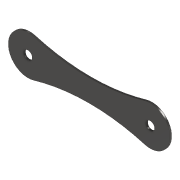
# Autodesk Inventor part: stelscharnier bovenkant
Saved by Autodesk Inventor 2020.3 (Build 243373000, 373)
## iProperties
Created: 2020-09-15
Part Number: stelscharnier bovenkant
Material: Stainless Steel
Document SubType Name: Modeling
Designer: Svend
Density: 8 g/cm^3
Appearance: Semi-Polished
Author: Svend
Autodesk Inventor part; units mm, degrees
ref_plane "YZ Plane" through (0, 0, 0) normal (1, 0, 0) x (0, 1, 0)
ref_plane "XZ Plane" through (0, 0, 0) normal (0, 1, 0) x (-1, 0, 0)
ref_plane "XY Plane" through (0, 0, 0) normal (0, 0, 1) x (1, 0, 0)
sketch "Sketch1" plane through (0, 0, 0) normal (0, 0, 1) x (1, 0, 0)
  circle A0 centre (0, 0) radius 22.5
  circle A1 centre (140, 0) radius 22.5
  arc A2 (6.3, 21.6) -> (133.7, 21.6) centre (70, 240) ccw
  line L0 (162.5, 0) -> (-22.5, 0) construction
  arc A3 (133.7, -21.6) -> (6.3, -21.6) centre (70, -240) ccw
  circle A4 centre (0, 0) radius 5
  circle A5 centre (140, 0) radius 5
  point P0 (70, 12.5)
  point P1 (6.3, -21.6)
  point P2 (133.7, -21.6)
  dimension "d0" = 45
  dimension "d1" = 140
  dimension "d2" = 12.5
  dimension "d3" = 10
  dimension "d4" = 10
  constraints: 9 point on circle, 6 centre point, 3 coincident, 3 symmetric about line, 2 end point, 2 tangent, 1 equal radius, 1 horizontal, 1 horizontal alignment, 1 point on line, 1 other
  measures "d0" diameter of A0
  measures "d1" distance of A0.centre A1.centre
  measures "d2" vertical distance of point (0, 0) point (70, 12.5)
  measures "d3" diameter of A4
  measures "d4" diameter of A5
extrude "Extrusion1" add sketch "Sketch1" along normal mid plane 2
body "Solid1"
